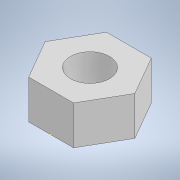
# Autodesk Inventor part: printCalibration
Saved by Autodesk Inventor 2020.3 (Build 243373000, 373)
## iProperties
Created: 2020-06-02
Part Number: printCalibration
Material: Generic
Document SubType Name: Modeling
Designer: robst
Density: 1 g/cm^3
Appearance: Default
Author: robst
Autodesk Inventor part; units mm, degrees
ref_plane "YZ Plane" through (0, 0, 0) normal (1, 0, 0) x (0, 1, 0)
ref_plane "XZ Plane" through (0, 0, 0) normal (0, 1, 0) x (-1, 0, 0)
ref_plane "XY Plane" through (0, 0, 0) normal (0, 0, 1) x (1, 0, 0)
sketch "Sketch1" plane through (0, 0, 0) normal (0, 1, 0) x (-1, 0, 0)
  line L0 (-14.6647, 0) -> (-7.3323, 12.7)
  line L1 (-7.3323, 12.7) -> (7.3323, 12.7)
  line L2 (7.3323, 12.7) -> (14.6647, 0)
  line L3 (14.6647, 0) -> (7.3323, -12.7)
  line L4 (7.3323, -12.7) -> (-7.3323, -12.7)
  line L5 (-7.3323, -12.7) -> (-14.6647, 0)
  circle A0 centre (0, 0) radius 6.35
  dimension "d0" = 25.4
  dimension "d1" = 12.7
  constraints: 12 end point, 2 coincident, 1 centre point, 1 horizontal, 13 other
  measures "d0" distance between parallel lines of L1 L4
  measures "d1" diameter of A0
extrude "Extrusion1" add sketch "Sketch1" along normal blind 12.7
sketch "Sketch2" plane through (-7.3323, 0, 12.7) normal (0, 0, 1) x (1, 0, 0)
  point P0 (7.3323, 0)
body "Solid1"
